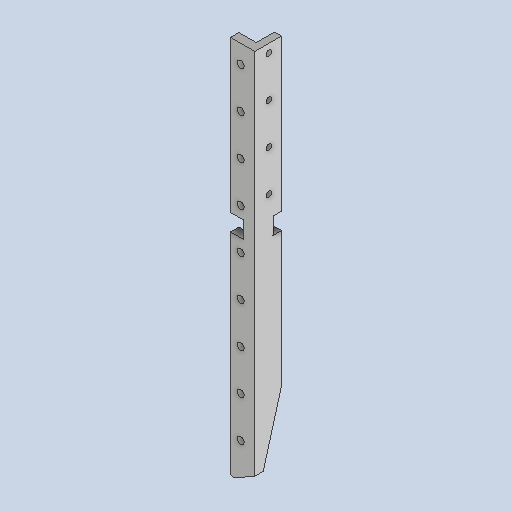
# Autodesk Inventor part: 1013
Saved by Autodesk Inventor 2025.1 (Build 291241000, 241)
## iProperties
Created: 2024-06-10
Part Number: 1013
Material: Generic
Document SubType Name: Modeling
Designer: Fabri
Density: 1 g/cm^3
Appearance: Default
Author: Fabri
Autodesk Inventor part; units mm, degrees
ref_plane "YZ Plane" through (0, 0, 0) normal (1, 0, 0) x (0, 1, 0)
ref_plane "XZ Plane" through (0, 0, 0) normal (0, 1, 0) x (-1, 0, 0)
ref_plane "XY Plane" through (0, 0, 0) normal (0, 0, 1) x (1, 0, 0)
sketch "Sketch1" plane through (0, 0, 0) normal (0, 1, 0) x (-1, 0, 0)
  line L0 (0, 0) -> (17.3205, 0)
  line L1 (0, -262) -> (0, 0)
  line L2 (17.3205, -272) -> (0, -262)
  line L3 (17.3205, -108) -> (8.3205, -108)
  line L4 (8.3205, -108) -> (8.3205, -120)
  line L5 (8.3205, -120) -> (17.3205, -120)
  line L6 (17.3205, 0) -> (17.3205, -108)
  line L7 (17.3205, -120) -> (17.3205, -272)
  dimension "d0" = 272
  dimension "d1" = 60
  dimension "d2" = 12
  dimension "d3" = 9
  dimension "d4" = 108
  dimension "d6" = 262
  constraints: 16 end point, 7 perpendicular, 2 parallel, 1 horizontal, 1 vertical alignment
  measures "d0" distance of L0.end L2.start
  measures "d1" angle of L1 L2
  measures "d2" distance between parallel lines of L5 L3
  measures "d3" distance between parallel lines of L4 L6
  measures "d4" distance from line of L3.start L0
  measures "d6" distance of L0.start L1.start
extrude "Extrusion1" add sketch "Sketch1" along normal mid plane 6
sketch "Sketch2" plane through (0, 3, 0) normal (0, 1, 0) x (1, 0, 0)
  line L0 (0, 0) -> (0, 262) projected
  point P0 (-10, 13)
  point P1 (-10, 42)
  point P2 (-10, 71)
  point P3 (-10, 100)
  point P4 (-10, 129)
  point P5 (-10, 158)
  point P6 (-10, 187)
  point P7 (-10, 216)
  point P8 (-10, 245)
  dimension "d9" = 10
  dimension "d10" = 17
  dimension "d11" = 13
  dimension "d12" = 29
  dimension "d13" = 29
  dimension "d14" = 29
  dimension "d15" = 29
  dimension "d16" = 29
  dimension "d17" = 29
  dimension "d18" = 29
  dimension "d19" = 29
  constraints: 8 vertical alignment
  measures "d9" distance from line of L0 point (-10, 13)
  measures "d10" vertical distance of point (-10, 245) L0.end
  measures "d11" vertical distance of point (-10, 13) L0.start
  measures "d12" distance of point (-10, 42) point (-10, 13)
  measures "d13" distance of point (-10, 71) point (-10, 42)
  measures "d14" distance of point (-10, 100) point (-10, 71)
  measures "d15" distance of point (-10, 129) point (-10, 100)
  measures "d16" distance of point (-10, 158) point (-10, 129)
  measures "d17" distance of point (-10, 187) point (-10, 158)
  measures "d18" distance of point (-10, 216) point (-10, 187)
  measures "d19" distance of point (-10, 245) point (-10, 216)
hole "Hole1" at (-10, 3, -13) at (-10, 3, -42) at (-10, 3, -71) at (-10, 3, -100) at (-10, 3, -129) at (-10, 3, -158) at (-10, 3, -187) at (-10, 3, -216) at (-10, 3, -245) direction (0, -1, 0) diameter 5 depth 6
sketch "Sketch3" plane through (0, 3, 0) normal (0, 1, 0) x (1, 0, 0)
  line L0 (0, 0) -> (-17.3205, 0) projected
  line L1 (0, 262) -> (0, 0) projected
  line L2 (-5, 0) -> (0, 0)
  line L3 (0, 0) -> (0, 262)
  line L4 (0, 262) -> (-5, 262)
  line L5 (-5, 262) -> (-5, 0)
  dimension "d27" = 5
  constraints: 8 end point, 2 parallel, 1 horizontal, 1 perpendicular, 1 point on line
  measures "d27" distance between parallel lines of L3 L5
extrude "Extrusion2" add sketch "Sketch3" along normal blind 13
sketch "Sketch4" plane through (-5, 3, -262) normal (-1, 0, 0) x (0, 0, 1)
  line L0 (0, 13) -> (262, 13) projected
  line L1 (154, 13) -> (154, 7)
  line L2 (154, 7) -> (142, 7)
  line L3 (142, 7) -> (142, 13)
  line L4 (262, 0) -> (262, 13) projected
  point P0 (262, -3)
  dimension "d30" = 12
  dimension "d31" = 6
  dimension "d32" = 108
  constraints: 6 end point, 3 perpendicular, 2 point on line
  measures "d30" distance of L1.end L2.end
  measures "d31" distance between parallel lines of L0 L2
  measures "d32" distance between parallel lines of L4 L1
extrude "Extrusion3" cut sketch "Sketch4" against normal blind 5
sketch "Sketch5" plane through (-5, 3, -262) normal (-1, 0, 0) x (0, 0, 1)
  line L0 (262, 0) -> (262, 13) projected
  line L1 (154, 13) -> (154, 7) projected
  line L2 (262, -6) -> (154, -6) projected
  point P0 (262, -3)
  point P1 (256, 4)
  point P2 (227, 4)
  point P3 (198, 4)
  point P4 (169, 4)
  point P5 (262, 6.5)
  dimension "d35" = 6
  dimension "d36" = 15
  dimension "d37" = 29
  dimension "d38" = 29
  dimension "d39" = 29
  dimension "d40" = 10
  constraints: 3 horizontal alignment, 1 midpoint
  measures "d35" horizontal distance of point (256, 4) point (262, 6.5)
  measures "d36" distance from line of L1 point (169, 4)
  measures "d37" distance of point (169, 4) point (198, 4)
  measures "d38" distance of point (198, 4) point (227, 4)
  measures "d39" distance of point (227, 4) point (256, 4)
  measures "d40" distance from line of L2 point (256, 4)
hole "Hole2" at (-5, 7, -6) at (-5, 7, -35) at (-5, 7, -64) at (-5, 7, -93) direction (1, 0, 0) diameter 4 depth 5 countersink diameter 5 countersink angle 90
sketch "Sketch6" plane through (-5, 3, -262) normal (-1, 0, 0) x (0, 0, 1)
  circle A0 centre (169, 4) radius 2.5 projected
  circle A1 centre (198, 4) radius 2.5 projected
  circle A2 centre (227, 4) radius 2.5 projected
  circle A3 centre (256, 4) radius 2.5 projected
  line L0 (154, 13) -> (154, 7) projected
  line L1 (154, 7) -> (142, 7) projected
  line L2 (142, 7) -> (142, 13) projected
  line L3 (0, 13) -> (142, 13) projected
  line L4 (0, 0) -> (0, 13) projected
  line L5 (262, 0) -> (0, 0) projected
  line L6 (262, 0) -> (262, 13) projected
  line L7 (154, 13) -> (262, 13) projected
  line L8 (0, 0) -> (46, 13)
  point P0 (262, -3)
  dimension "d48" = 96
  constraints: 2 end point, 1 point on line
  measures "d48" distance from line of L8.end L2
extrude "Extrusion4" cut sketch "Sketch6" against normal up to surface (5 mm away) contours L4 L3 L8
fillet "Fillet1" radius 2 1 edges at (-17.3205, 0, -272)
equation "\"d13\" = d12"
equation "\"d14\" = d12"
equation "\"d15\" = d12"
equation "\"d16\" = d12"
equation "\"d17\" = d12"
equation "\"d18\" = d12"
equation "\"d38\" = d37"
body "Solid1"
